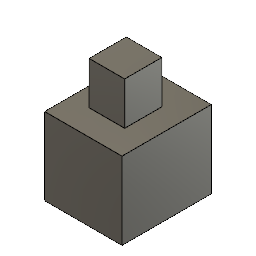
switch (Autodesk Fusion 360 design; units mm, degrees)
Autodesk Fusion 360 part; units mm, degrees
sketch "Sketch1" plane through (0, 0, 0) normal (0, 1, 0) x (1, 0, 0)
  line L0 (0, 0) -> (2.9, 0)
  line L1 (2.9, 0) -> (2.9, -3.35)
  line L2 (2.9, -3.35) -> (0, -3.35)
  line L3 (0, -3.35) -> (0, 0)
  dimension "d1" = 3.35
  dimension "d2" = 2.9
  measures "d1" distance of L0.start L2.end
  measures "d2" distance of L1.end L2.end
extrude "Extrude1" add sketch "Sketch1" along normal blind 2.9
sketch "Sketch2" plane through (0, 2.9, 0) normal (0, 1, 0) x (-1, 0, 0)
  line L0 (0, 3.35) -> (-2.9, 3.35)
  line L1 (-2.9, 3.35) -> (-2.9, 0)
  line L2 (-2.9, 0) -> (0, 0)
  line L3 (0, 0) -> (0, 3.35)
  line L4 (-0.712, 0.999) -> (-2.047, 0.999)
  line L5 (-2.047, 0.999) -> (-2.047, 2.397)
  line L6 (-2.047, 2.397) -> (-0.712, 2.397)
  line L7 (-0.712, 2.397) -> (-0.712, 0.999)
  dimension "d5" = 1.398
  dimension "d6" = 1.335
  dimension "d7" = 0.953
  dimension "d8" = 0.712
  measures "d5" distance of L4.start L6.end
  measures "d6" distance of L5.end L6.end
  measures "d7" distance of L0 L6
  measures "d8" distance of L3 L7
extrude "Extrude2" add sketch "Sketch2" along normal blind 1.6 contours L4 L5 L6 L7
